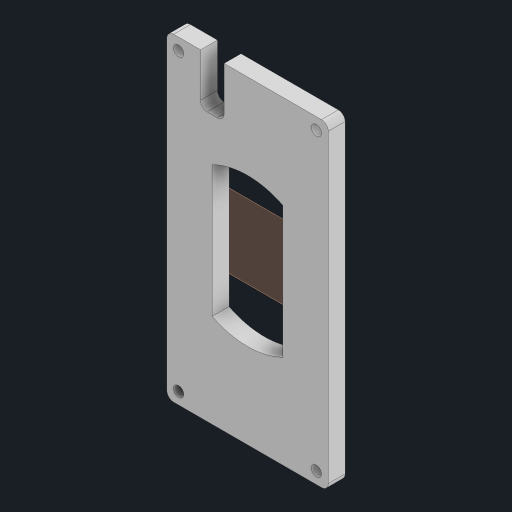
# Autodesk Inventor part: TAPA_CAMARA_2
Saved by Autodesk Inventor 2024.3 (Build 283343000, 343)
## iProperties
Created: 2024-07-21
Part Number: TAPA_CAMARA_2
Material: Generic
Document SubType Name: Modeling
Designer: Niler
Density: 1 g/cm^3
Appearance: Default
Author: Niler
Autodesk Inventor part; units mm, degrees
ref_plane "YZ Plane" through (0, 0, 0) normal (1, 0, 0) x (0, 1, 0)
ref_plane "XZ Plane" through (0, 0, 0) normal (0, 1, 0) x (-1, 0, 0)
ref_plane "XY Plane" through (0, 0, 0) normal (0, 0, 1) x (1, 0, 0)
ref_plane "Work Plane1" through (-23.955, 47.3, 0) normal (0, 0, 1) x (0, -1, 0)
sketch "Sketch1" plane through (-23.955, 47.3, 0) normal (0, 0, 1) x (0, -1, 0)
  arc A0 (2, 47.9099) -> (0, 45.9099) centre (2, 45.9099) ccw projected
  line L0 (0, 45.9099) -> (0, 2) projected
  arc A1 (0, 2) -> (2, 0) centre (2, 2) ccw projected
  line L1 (2, 0) -> (92.6, 0) projected
  arc A2 (92.6, 0) -> (94.6, 2) centre (92.6, 2) ccw projected
  line L2 (94.6, 2) -> (94.6, 45.9099) projected
  arc A3 (94.6, 45.9099) -> (92.6, 47.9099) centre (92.6, 45.9099) ccw projected
  line L3 (92.6, 47.9099) -> (2, 47.9099) projected
  line L4 (7, 7) -> (7, 40.9099) projected
  line L5 (7, 40.9099) -> (87.6, 40.9099) projected
  line L6 (87.6, 40.9099) -> (87.6, 7) projected
  line L7 (87.6, 7) -> (7, 7) projected
  circle A4 centre (91.1, 3.5) radius 1.5 projected
  circle A5 centre (3.5, 3.5) radius 1.5 projected
  circle A6 centre (91.1, 44.4099) radius 1.5 projected
  circle A7 centre (3.5, 44.4099) radius 1.5 projected
  point P0 (47.3, 23.955)
extrude "Extrusion1" add sketch "Sketch1" along normal blind 5 contours L3 A3 L2 A2 L1 A1 L0 A0 | L4 L5 L6 L7
sketch "Sketch2" plane through (-23.955, 47.3, 5) normal (0, 0, 1) x (1, 0, 0)
  line L0 (13.455, -25.3) -> (34.455, -25.3)
  line L1 (34.455, -25.3) -> (34.455, -69.3)
  line L2 (34.455, -69.3) -> (13.455, -69.3)
  line L3 (13.455, -69.3) -> (13.455, -25.3)
  line L4 (13.455, -25.3) -> (34.455, -69.3) construction
  line L5 (34.455, -25.3) -> (13.455, -69.3) construction
  line L6 (34.455, -27.8) -> (13.455, -27.8)
  arc A0 (34.455, -27.8) -> (13.455, -27.8) centre (23.955, -48.6) ccw
  line L7 (45.9099, 0) -> (2, 0) projected
  arc A1 (2, 0) -> (0, -2) centre (2, -2) ccw projected
  line L8 (0, -2) -> (0, -92.6) projected
  arc A2 (0, -92.6) -> (2, -94.6) centre (2, -92.6) ccw projected
  line L9 (2, -94.6) -> (45.9099, -94.6) projected
  arc A3 (45.9099, -94.6) -> (47.9099, -92.6) centre (45.9099, -92.6) ccw projected
  line L10 (47.9099, -92.6) -> (47.9099, -2) projected
  arc A4 (47.9099, -2) -> (45.9099, 0) centre (45.9099, -2) ccw projected
  circle A5 centre (44.4099, -3.5) radius 1.5 projected
  circle A6 centre (44.4099, -91.1) radius 1.5 projected
  circle A7 centre (3.5, -3.5) radius 1.5 projected
  circle A8 centre (3.5, -91.1) radius 1.5 projected
  line L11 (47.9099, -47.3) -> (0, -47.3)
  line L12 (0, -2) -> (0, -92.6) projected
  arc A9 (13.455, -66.8) -> (34.455, -66.8) centre (23.955, -46) ccw
  point P0 (23.955, -47.3)
  point P1 (23.955, -25.3)
  point P2 (13.455, -66.8)
  point P3 (34.455, -66.8)
  dimension "d2" = 21
  dimension "d3" = 44
  dimension "d4" = 2.5
  constraints: 16 end point, 5 midpoint, 5 point on circle, 3 symmetric about line, 2 centre point, 2 parallel, 2 perpendicular, 2 point on line, 1 horizontal, 1 other
  measures "d2" distance of L1.end L2.end
  measures "d3" distance of L0.end L1.end
  measures "d4" distance between parallel lines of L0 L6
extrude "Extrusion2" cut sketch "Sketch2" against normal through all contours A0 L6 | L6 L1 L11 L3 | L11 L1 A9 L3
sketch "Sketch3" plane through (-23.955, 47.3, 0) normal (0, 0, -1) x (-1, 0, 0)
  arc A0 (-34.455, -66.8) -> (-13.455, -66.8) centre (-23.955, -46) ccw projected
  line L0 (-34.455, -66.8) -> (-34.455, -27.8) projected
  arc A1 (-13.455, -27.8) -> (-34.455, -27.8) centre (-23.955, -48.6) ccw projected
  line L1 (-13.455, -27.8) -> (-13.455, -66.8) projected
  line L2 (-45.9099, 0) -> (-2, 0) projected
  arc A2 (-45.9099, 0) -> (-47.9099, -2) centre (-45.9099, -2) ccw projected
  line L3 (-47.9099, -92.6) -> (-47.9099, -2) projected
  arc A3 (-47.9099, -92.6) -> (-45.9099, -94.6) centre (-45.9099, -92.6) ccw projected
  line L4 (-2, -94.6) -> (-45.9099, -94.6) projected
  arc A4 (-2, -94.6) -> (0, -92.6) centre (-2, -92.6) ccw projected
  line L5 (0, -2) -> (0, -92.6) projected
  arc A5 (0, -2) -> (-2, 0) centre (-2, -2) ccw projected
  circle A6 centre (-44.4099, -3.5) radius 1.5 projected
  circle A7 centre (-44.4099, -91.1) radius 1.5 projected
  circle A8 centre (-3.5, -3.5) radius 1.5 projected
  circle A9 centre (-3.5, -91.1) radius 1.5 projected
  line L6 (-17, 0) -> (-10, 0)
  line L7 (-10, 0) -> (-10, -12.9385)
  line L8 (-12, -14.9385) -> (-15, -14.9385)
  line L9 (-17, -12.9385) -> (-17, 0)
  arc A10 (-17, -12.9385) -> (-15, -14.9385) centre (-15, -12.9385) ccw
  arc A11 (-12, -14.9385) -> (-10, -12.9385) centre (-12, -12.9385) ccw
  line L10 (-10, -7) -> (-17, -7)
  point P0 (-23.955, -47.3)
  point P1 (-10, -14.9385)
  point P2 (-17, -14.9385)
  point P3 (-10, 0)
  dimension "d7" = 7
  dimension "d9" = 2
  dimension "d12" = 10
  dimension "d13" = 7
  constraints: 10 end point, 7 point on line, 4 point on circle, 4 tangent, 2 centre point, 2 parallel, 2 perpendicular, 1 equal radius, 1 horizontal
  measures "d7" distance of point (-10, -14.938) point (-17, -14.938)
  measures "d9" radius of A10
  measures "d12" distance between parallel lines of L5 L7
  measures "d13" distance between parallel lines of L2 L10
extrude "Extrusion3" cut sketch "Sketch3" against normal through all contours L2 L7 L10 L9 | L10 L7 A11 L8 A10 L9
body "Solid1"
